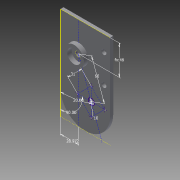
# Autodesk Inventor part: plate_bot
Saved by Autodesk Inventor 2015 SP2 (Build 190223200, 223)
## iProperties
Created: 2016-03-07
Part Number: plate_bot
Material: Generic
Document SubType Name: Modeling
Designer: marc
Density: 1 g/cm^3
Appearance: Default
Author: marc
Autodesk Inventor part; units mm, degrees
ref_plane "YZ Plane" through (0, 0, 0) normal (1, 0, 0) x (0, 1, 0)
ref_plane "XZ Plane" through (0, 0, 0) normal (0, 1, 0) x (-1, 0, 0)
ref_plane "XY Plane" through (0, 0, 0) normal (0, 0, 1) x (1, 0, 0)
sketch "Sketch1" plane through (0, 0, 0) normal (0, 1, 0) x (-1, 0, 0)
  line L0 (0, 0) -> (80, 0)
  line L1 (80, 0) -> (80, -150)
  line L2 (80, -150) -> (0, -150)
  line L3 (0, -150) -> (0, 0)
  dimension "d0" = 150
  dimension "d1" = 80
  constraints: 8 end point, 2 parallel, 1 horizontal, 1 perpendicular
  measures "d0" distance of L2.end L0.start
  measures "d1" distance between parallel lines of L1 L3
extrude "Extrusion1" add sketch "Sketch1" along normal blind 5
sketch "Sketch3" plane through (0, 0, 0) normal (0, -1, 0) x (1, 0, 0)
  line L0 (-80, 0) -> (0, 0) construction
  line L1 (0, -150) -> (-80, -150) construction
  line L2 (-51.028, -150) -> (-51.028, 0) construction
  line L3 (-80, 0) -> (-80, -150) projected
  point P0 (-51.028, -48)
  dimension "PusherHoleOffset" = 28.972
  dimension "d56" = 48
  constraints: 3 point on line, 2 end point, 1 perpendicular
  measures "PusherHoleOffset" distance between parallel lines of L3 L2
  measures "d56" distance from line of L0 point (-51.028, -48)
hole "Hole2" at (-51.028, 0, -48) direction (0, 1, 0) diameter 9 end through all clearance for "Socket Head Cap Screw ISO 4762" size "M8" standard "ISO"
sketch "Sketch6" plane through (0, 0, 0) normal (0, -1, 0) x (1, 0, 0)
  line L0 (-80, 0) -> (0, 0) construction
  line L1 (0, -150) -> (-80, -150) construction
  circle A0 centre (-51.028, -48) radius 11
  circle A1 centre (-51.028, -48) radius 16
  line L2 (-51.028, -150) -> (-51.028, 0) construction
  line L3 (-80, -150) -> (-80, 0) construction
  dimension "bearingOD" = 22
  dimension "d38" = 5
  dimension "d53" = 28.972
  dimension "d57" = 48
  constraints: 3 point on line, 2 centre point, 2 end point, 1 coincident, 1 perpendicular
  measures "bearingOD" diameter of A0
  measures "d38" radial gap between concentric circles of A1 A0
  measures "d53" distance between parallel lines of L3 L2
  measures "d57" distance from line of L0 A1.centre
extrude "Extrusion3" add sketch "Sketch6" along normal blind 7
sketch "Sketch7" plane through (0, 0, 0) normal (0, -1, 0) x (1, 0, 0)
  line L0 (-10, -71) -> (-10, -25) construction
  line L1 (0, -150) -> (0, 0) construction
  line L2 (0, 0) -> (-80, 0) construction
  dimension "rodDistFromEdge" = 10
  dimension "OffsetSupportRod" = 25
  dimension "DistSupportRod" = 46
  constraints: 2 end point, 1 vertical
  measures "rodDistFromEdge" distance between parallel lines of L1 L0
  measures "OffsetSupportRod" distance from line of L2 L0.end
  measures "DistSupportRod" distance of L0.end L0.start
hole "Hole4" at (-10, 0, -71) at (-10, 0, -25) direction (0, 1, 0) diameter 8 end through all
sketch "Sketch8" plane through (0, 0, 0) normal (0, -1, 0) x (1, 0, 0)
  circle A0 centre (-51.028, -48) radius 4.5 construction
  line L0 (-51.028, -48) -> (-12.9125, -152.7215) construction
  line L1 (0, 0) -> (-80, 0) construction
  line L2 (0, -150) -> (-80, -150) construction
  line L3 (-80, 0) -> (-80, -150) construction
  line L4 (-30.5068, -82.4612) -> (-8.5865, -104.3816) construction
  line L5 (-8.5865, -104.3816) -> (-30.5068, -126.3019) construction
  line L6 (-30.5068, -126.3019) -> (-52.4271, -104.3816) construction
  line L7 (-52.4271, -104.3816) -> (-30.5068, -82.4612) construction
  line L8 (-8.5865, -104.3816) -> (-52.4271, -104.3816) construction
  line L9 (-30.5068, -82.4612) -> (-30.5068, -126.3019) construction
  circle A1 centre (-30.5068, -104.3816) radius 5
  dimension "d58" = 20
  dimension "d59" = 31
  dimension "d60" = 60
  dimension "d62" = 90
  dimension "d70" = 10
  constraints: 14 end point, 5 coincident, 3 perpendicular, 1 centre point, 1 midpoint, 1 parallel, 1 point on line
  measures "d58" angle of L3 L0
  measures "d59" distance of L6.end L4.start
  measures "d60" distance of L0.start point (-30.507, -104.382)
  measures "d62" angle of L8 L3
  measures "d70" diameter of A1
hole "Hole5" at (-30.5068, 0, -126.3019) at (-52.4271, 0, -104.3816) at (-30.5068, 0, -82.4612) at (-8.5865, 0, -104.3816) direction (0, 1, 0) diameter 3.4 end through all clearance for "Socket Head Cap Screw ISO 4762" size "M3" standard "ISO"
extrude "Extrusion4" cut sketch "Sketch8" against normal through all
fillet "Fillet1" radius 40 2 edges at (0, 2.5, -150) (-80, 2.5, -150)
equation "\"d56\" = OffsetSupportRod + 0.5 * DistSupportRod"
equation "\"d53\" = holeOffsetP"
equation "\"d57\" = d56"
equation "\"holeOffsetP\" = 28.972"
body "Solid1"
